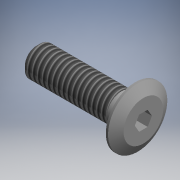
# Autodesk Inventor part: CBSTSR3-10
Saved by Autodesk Inventor 2017.3 (Build 213256000, 256)
## iProperties
Part Number: CBSTSR3-10
Material: Generic
Catalog Web Link: www.cadenas.de
Description: CBSTSR,CBSTBR,CBSTNR-Ultra Low Head Cap Screws - Hex Sockets
Vendor: MISUMI
Document SubType Name: Modeling
Designer: partserver
Manufacturer: MISUMI
Mass: 0.0823399 g
Surface Area: 1.66384 cm^2
Volume: 0.0823399 cm^3
Density: 1 g/cm^3
Appearance: PSOLRGB-175-175-175
Category: PARTsolutions
Company: MISUMI
Title: CBSTSR3-10
Author: Cadenas PARTsolutions
Comments: Ultra Low Head Cap Screws - Hex Sockets
PSOL_IDENT_0: {$CADENAS_DATA\23d-libs\misumi\metric\27_screws_nuts\cbstsr.prj},183 {VTYP=3D},{NB=CBSTSR3-10},{LINA=
PSOL_IDENT_1: CBSTSR3-10},{NN=CBSTSR,CBSTBR,CBSTNR},{DATE=03.06.2021 03:35:26},{GEOMDATE=04.03.2020 04:03:33},{VER
PSOL_IDENT_2: SION=},{LINEID=60},{WBVAR=MAT,ST,L},{WBNUMERIC=L}  {NB=CBSTSR3-10},{LINA=CBSTSR3-10},{KT=DUMMY},{PN=
PSOL_IDENT_3: CBSTSR3-10},{TYPE=CBSTSR},{MAT=SUS304},{HARD=-},{ST=-},{STALG='-','-'},{STPN=},{M=3.0},{L=10},{LALG=
PSOL_IDENT_4: 4,5,6,8,10,12,14,16},{LS=4,5,6,8,10,12,14,16},{LNB=4,5,6,8,10,12,16},{P=0.50},{MP=M3x0.5},{A=6},{B=1
PSOL_IDENT_5: .5},{E=0.8},{TT=2.0},{EE=1.4},{RR=0.10},{AA=1}
NB: CBSTSR3-10
NN: CBSTSR,CBSTBR,CBSTNR
NT: Ultra Low Head Cap Screws - Hex Sockets
NBSYN: $PN.
LINA: CBSTSR3-10
CATALOG: Misumi
PN: CBSTSR3-10
TYPE: CBSTSR
MAT: 304 Stainless Steel
HARD: -
ST: -
M: 3
L: 10
LS: 4,5,6,8,10,12,14,16
LNB: 4,5,6,8,10,12,16
MP: M3x0.5
A: 6
B: 1.5
E: 0.8
TT: 2
EE: 1.4
RR: 0.1
SUPPLIER: MISUMI
ARTICLENO: CBSTSR3-10
BOMINFO: CBSTSR3-10
CREATOR: CADENAS GmbH
Autodesk Inventor part; units mm, degrees
ref_plane "YZ Plane" through (0, 0, 0) normal (1, 0, 0) x (0, 1, 0)
ref_plane "XZ Plane" through (0, 0, 0) normal (0, 1, 0) x (-1, 0, 0)
ref_plane "XY Plane" through (0, 0, 0) normal (0, 0, 1) x (1, 0, 0)
sketch "Sketch_1" plane through (0, 0, 0) normal (0, 0, 1) x (1, 0, 0)
  line L0 (10, 0) -> (-0.8, 0)
  line L1 (-0.8, 0) -> (-0.8, 2)
  line L2 (-0.8, 2) -> (-0.2226, 3)
  line L3 (-0.2226, 3) -> (0, 3)
  line L4 (0, 3) -> (0, 1.4467)
  arc A0 (0, 1.4467) -> (0.1, 1.3467) centre (0.1, 1.4467) ccw
  line L5 (0.1, 1.3467) -> (0.9, 1.3467)
  line L6 (0.9, 1.3467) -> (1.4, 1.5)
  line L7 (1.4, 1.5) -> (9.6935, 1.5)
  line L8 (9.6935, 1.5) -> (10, 1.1935)
  line L9 (10, 1.1935) -> (10, 0)
  line L10 (10, 0) -> (-0.8, 0)
  constraints: 22 end point, 2 point on circle, 1 centre point
revolve "Revolution1" add sketch "Sketch_1" angle 360 about axis through (10, 0, 0) along (1, 0, 0)
thread "Thread1" size "M3x0.5" class "6g" standard "ISO Metric profile" full length
sketch "Sketch2" plane through (-0.8, 0, 0) normal (-1, 0, 0) x (0, 0, 1)
  point P0 (0, 0)
hole "Hole1" at (-0.8, 0, 0) direction (1, 0, 0) diameter 1.5 depth 2 tip angle 120
sketch "Sketch_3" plane through (-0.8, 0, 0) normal (1, 0, 0) x (0, 0, -1)
  line L0 (-0.75, -0.433) -> (0, -0.866)
  line L1 (0, -0.866) -> (0.75, -0.433)
  line L2 (0.75, -0.433) -> (0.75, 0.433)
  line L3 (0.75, 0.433) -> (0, 0.866)
  line L4 (0, 0.866) -> (-0.75, 0.433)
  line L5 (-0.75, 0.433) -> (-0.75, -0.433)
  constraints: 12 end point
extrude "Extrusion1" cut sketch "Sketch_3" along normal blind 2
body "Solid1"
